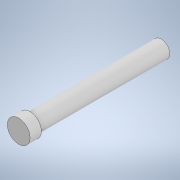
# Autodesk Inventor part: CilindroHidraulico_2
Saved by Autodesk Inventor 2021 (Build 250183000, 183)
## iProperties
Created: 2021-07-12
Part Number: CilindroHidraulico_2
Material: Generic
Document SubType Name: Modeling
Designer: Nelson
Density: 1 g/cm^3
Appearance: Default
Author: Nelson
Autodesk Inventor part; units mm, degrees
ref_plane "YZ Plane" through (0, 0, 0) normal (1, 0, 0) x (0, 1, 0)
ref_plane "XZ Plane" through (0, 0, 0) normal (0, 1, 0) x (-1, 0, 0)
ref_plane "XY Plane" through (0, 0, 0) normal (0, 0, 1) x (1, 0, 0)
sketch "Sketch3" plane through (0, 0, 0) normal (1, 0, 0) x (0, 1, 0)
  line L0 (0, 0) -> (37.5, 0)
  line L1 (0, 0) -> (0, -37)
  line L2 (0, -37) -> (9.5, -37)
  line L3 (9.5, -37) -> (9.5, -469)
  line L4 (37.5, 0) -> (37.5, -469)
  line L5 (37.5, -469) -> (9.5, -469)
  dimension "d3" = 37.5
  dimension "d4" = 37
  dimension "d8" = 28
  dimension "d10" = 469
  constraints: 12 end point, 3 vertical, 2 horizontal, 1 perpendicular
  measures "d3" distance of L0.start L0.end
  measures "d4" distance of L0.start L1.end
  measures "d8" distance of L4.end L3.end
  measures "d10" distance of L0.end L4.end
revolve "Revolution1" add sketch "Sketch3" angle 360 about axis through (0, 37.5, 0) along (0, 0, -1)
body "Solid1"
